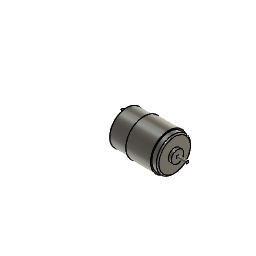
salvagev2 (Autodesk Fusion 360 design; units mm, degrees)
Autodesk Fusion 360 part; units mm, degrees
sketch "Sketch1" plane through (0, 0, 0) normal (0, 1, 0) x (1, 0, 0)
  line L0 (0, 0) -> (37.7, 0)
  line L1 (37.7, 0) -> (37.7, -13.75)
  line L2 (37.7, -13.75) -> (0, -13.75)
  line L3 (0, -13.75) -> (0, 0)
  line L4 (37.7, -5) -> (40.1, -5)
  line L5 (40.1, -5) -> (40.1, 0)
  line L6 (40.1, 0) -> (37.7, 0)
  line L7 (37.7, 0) -> (37.7, -5)
  line L8 (40.1, -1.05) -> (47.9, -1.05)
  line L9 (47.9, -1.05) -> (47.9, 0)
  line L10 (47.9, 0) -> (40.1, 0)
  line L11 (40.1, 0) -> (40.1, -1.05)
  line L12 (0, -5) -> (-2.5, -5)
  line L13 (-2.5, -5) -> (-2.5, 0)
  line L14 (-2.5, 0) -> (0, 0)
  line L15 (0, 0) -> (0, -5)
  line L16 (13, -13.75) -> (33, -13.75)
  line L17 (33, -13.75) -> (33, -14.75)
  line L18 (33, -14.75) -> (13, -14.75)
  line L19 (13, -14.75) -> (13, -13.75)
  dimension "d74" = 37.7
  dimension "d75" = 20
  dimension "d76" = 2.4
  dimension "d77" = 7.8
  dimension "d78" = 1.05
  dimension "d79" = 5
  dimension "d80" = 13.75
  dimension "d81" = 1
  dimension "d82" = 5
  dimension "d83" = 2.5
  dimension "d84" = 13
  constraint horizontal L0
  constraint vertical L1
  constraint horizontal L2
  constraint vertical L3
  constraint coincident L0.start L3.end
  constraint horizontal L4
  constraint vertical L5
  constraint horizontal L6
  constraint vertical L7
  constraint coincident L1 L4.start
  constraint horizontal L8
  constraint vertical L9
  constraint horizontal L10
  constraint vertical L11
  constraint coincident L5 L8.start
  constraint horizontal L12
  constraint vertical L13
  constraint horizontal L14
  constraint vertical L15
  constraint coincident L3 L12.start
  constraint horizontal L16
  constraint vertical L17
  constraint horizontal L18
  constraint vertical L19
  constraint coincident L2 L16.start
  constraint collinear L0 L14
  constraint collinear L0 L6
  constraint collinear L6 L10
  measures "d74" distance of L1.end L2.end
  measures "d75" distance of L17.end L18.end
  measures "d76" distance of L4.start L4.end
  measures "d77" distance of L8.start L8.end
  measures "d78" distance of L8.end L9.end
  measures "d79" distance of L4.end L5.end
  measures "d80" distance of L0.end L1.end
  measures "d81" distance of L16.end L17.end
  measures "d82" distance of L12.end L13.end
  measures "d83" distance of L12.start L12.end
  measures "d84" distance of L2.end L16.start
revolve "Revolve1" add sketch "Sketch1" angle 360 about axis through (0, 0, 0) along (1, 0, 0)
sketch "Sketch2" plane through (-2.5, 0, 0) normal (-1, 0, 0) x (0, -1, 0)
  circle A0 centre (0, 0) radius 5
  circle A1 centre (0, 0) radius 4.25
  dimension "d86" = -0.75
extrude "Extrude1" cut sketch "Sketch2" against normal blind 0.75 contours A1
sketch "Sketch3" plane through (-1.75, 0, 0) normal (-1, 0, 0) x (0, -1, 0)
  circle A0 centre (0, 0) radius 4.25
  circle A1 centre (0, 0) radius 1.125
  dimension "d89" = 2.25
  constraint concentric A0 A1
  measures "d89" diameter of A1
extrude "Extrude2" add sketch "Sketch3" along normal blind 1 contours A1
fillet "Fillet1" radius 0.25 1 edges at (-2.75, 1.0489, -0.4068)
fillet "Fillet2" radius 1 1 edges at (37.7, -4.9722, -12.8195)
sketch "Sketch4" plane through (0, 0, 0) normal (-1, 0, 0) x (0, -1, 0)
  circle A0 centre (0, 0) radius 13.75
  circle A1 centre (0, 0) radius 5
  circle A2 centre (0, 0) radius 13
  dimension "d96" = -0.75
extrude "Extrude3" add sketch "Sketch4" along normal blind 1 contours A0
sketch "Sketch6" plane through (0, 0, 0) normal (-1, 0, 0) x (0, -1, 0)
  circle A0 centre (0, 0) radius 13
  circle A1 centre (0, 0) radius 5
  line L0 (-1.9987, 12) -> (2.0013, 12)
  line L1 (2.0013, 12) -> (2.0013, 10)
  line L2 (2.0013, 10) -> (-1.9987, 10)
  line L3 (-1.9987, 10) -> (-1.9987, 12)
  line L4 (-1.9987, -10) -> (2.0013, -10)
  line L5 (2.0013, -10) -> (2.0013, -12)
  line L6 (2.0013, -12) -> (-1.9987, -12)
  line L7 (-1.9987, -12) -> (-1.9987, -10)
  line L8 (0.0013, 10) -> (0.0013, -10)
  dimension "d101" = 4
  dimension "d102" = 2
  dimension "d103" = 10
  dimension "d104" = 10
  constraint horizontal L0
  constraint vertical L1
  constraint horizontal L2
  constraint vertical L3
  constraint horizontal L4
  constraint vertical L5
  constraint horizontal L6
  constraint vertical L7
  constraint collinear L1 L5
  constraint equal L0 L4
  constraint equal L1 L5
  constraint midpoint L2 L8.start
  constraint midpoint L4 L8.end
  measures "d101" distance of L0.start L0.end
  measures "d102" distance of L0.end L1.end
  measures "d103" vertical distance of A0.centre L8.start
  measures "d104" vertical distance of A0.centre L8.end
extrude "Extrude4" add sketch "Sketch6" along normal blind 1 contours L0 L1 L2 L3 | L4 L5 L6 L7
sketch "Sketch7" plane through (-1, 0, 0) normal (-1, 0, 0) x (0, -1, 0)
  line L0 (-1.9987, -12) -> (2.0013, -12)
  line L1 (2.0013, -12) -> (2.0013, -10)
  line L2 (2.0013, -10) -> (-1.9987, -10)
  line L3 (-1.9987, -10) -> (-1.9987, -12)
  line L4 (-1, -11) -> (1, -11)
  line L5 (1, -11) -> (1, -11.5)
  line L6 (1, -11.5) -> (-1, -11.5)
  line L7 (-1, -11.5) -> (-1, -11)
  line L8 (-1, 11) -> (1, 11)
  line L9 (1, 11) -> (1, 10.5)
  line L10 (1, 10.5) -> (-1, 10.5)
  line L11 (-1, 10.5) -> (-1, 11)
  constraint horizontal L4
  constraint vertical L5
  constraint horizontal L6
  constraint vertical L7
  constraint horizontal L8
  constraint vertical L9
  constraint horizontal L10
  constraint vertical L11
extrude "Extrude5" add sketch "Sketch7" along normal blind 4 contours L4 L5 L6 L7 | L8 L9 L10 L11
fillet "Fillet3" radius 0.5 4 edges at (-5, 1, 10.75) (-5, -1, 10.75) (-5, -1, -11.25) (-5, 1, -11.25)
equation "d78 = ( 2.1 / 2 ) * 1 mm"
equation "d80 = ( 27.5 / 2 ) * 1 mm"
